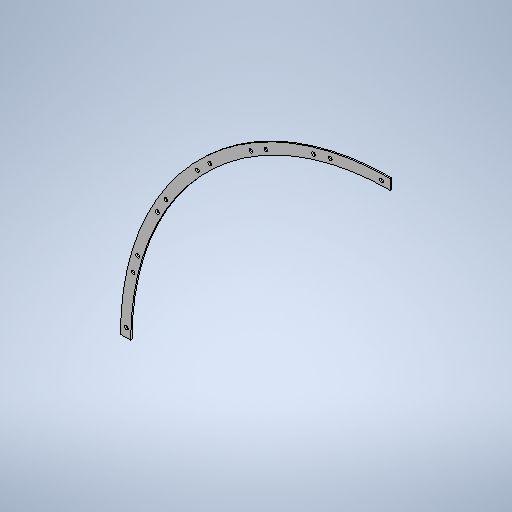
# Autodesk Inventor part: DMF 2.1 01 43 Gear rim 3_CPY
Saved by Autodesk Inventor 2026.2 (Build 302298010, 298A)
## iProperties
Created: 2024-04-30
Part Number: DMF 2.1 01 43 Gear rim 3_CPY
Material: Stainless Steel
Document SubType Name: Sheet Metal
Designer: admin
Stock Number: Барабан_Сектор_Усилителя
Mass: 2673.55 g
Surface Area: 3449.14 cm^2
Volume: 334.194 cm^3
Density: 8 g/cm^3
Flat Pattern Width: 58 cm
Flat Pattern Length: 58 cm
Flat Pattern Area: 3364 cm^2
Sheet Metal Rule: Default
Sheet Metal Width: 580,000 mm
Sheet Metal Length: 580,000 mm
Sheet Metal Area: 336400,000 mm^2
Appearance: Default
Author: pokla
Autodesk Inventor part; units mm, degrees
ref_plane "YZ Plane" through (0, 0, 0) normal (1, 0, 0) x (0, 1, 0)
ref_plane "XZ Plane" through (0, 0, 0) normal (0, 1, 0) x (-1, 0, 0)
ref_plane "XY Plane" through (0, 0, 0) normal (0, 0, 1) x (1, 0, 0)
sketch "Sketch1" plane through (0, 0, 0) normal (0, 0, 1) x (1, 0, 0)
  circle A0 centre (0, 0) radius 558
  circle A1 centre (0, 0) radius 580
  line L0 (0, 0) -> (-580, 0)
  line L1 (0, 0) -> (0, 580) construction
  line L2 (0, 0) -> (0, 580)
  circle A2 centre (0, 0) radius 100
  line L3 (197.082, 197.082) -> (278.716, 0)
  line L4 (278.716, 0) -> (197.082, -197.082)
  line L5 (197.082, -197.082) -> (0, -278.716)
  line L6 (0, -278.716) -> (-197.082, -197.082)
  line L7 (-197.082, -197.082) -> (-278.716, 0)
  line L8 (-278.716, 0) -> (-197.082, 197.082)
  line L9 (-197.082, 197.082) -> (0, 278.716)
  line L10 (0, 278.716) -> (197.082, 197.082)
  point P0 (-558, 0)
  point P1 (0, 558)
  point P2 (-100, 0)
  point P3 (0, 100)
  point P4 (0, 278.716)
  point P5 (-278.716, 0)
  dimension "d30" = 90
  dimension "d31" = 1160
  dimension "d32" = 1116
  dimension "d65" = 90
  dimension "d66" = 200
  dimension "d91" = 515
  measures "d30" angle of L2 L0
  measures "d31" diameter of A1
  measures "d32" diameter of A0
  measures "d65" angle of L1 L0
  measures "d66" diameter of A2
  measures "d91" distance between parallel lines of L5 L9
extrude "Plate1" add sketch "Sketch1" against normal blind 3 contours A0 L0 A1 L2 picked at (-572.0249, 22.0563)
sketch "Sketch2" plane through (0, 0, 0) normal (0, 0, 1) x (1, 0, 0)
  circle A0 centre (0, 0) radius 567.5
  arc A1 (0, 580) -> (-580, 0) centre (0, 0) ccw projected
  line L0 (0, 0) -> (0, 580) construction
  line L1 (0, 0) -> (-18.5681, 567.1962) construction
  line L2 (-128.8658, 552.6752) -> (0, 0) construction
  line L3 (0, 0) -> (0, 567.5) construction
  line L4 (0, 0) -> (18.5681, 567.1962) construction
  line L5 (0, 0) -> (128.8658, 552.6752) construction
  line L6 (0, 0) -> (-164.7366, 543.0636) construction
  line L7 (0, 0) -> (-267.5176, 500.4903) construction
  dimension "d34" = 1135
  dimension "d35" = 1.875
  dimension "d36" = 11.25
  dimension "d44" = 1.875
  dimension "d45" = 11.25
  dimension "d49" = 3.75
  dimension "d50" = 11.25
  constraints: 16 end point, 3 coincident, 1 vertical, 9 other
  measures "d35" angle of L0 L1
  measures "d36" angle of L1 L2
  measures "d44" angle of L4 L3
  measures "d45" angle of L5 L4
  measures "d49" angle of L2 L6
  measures "d50" angle of L6 L7
hole "Hole1" at (-18.5681, 567.1962, 0) at (-128.8658, 552.6752, 0) at (128.8658, 552.6752, 0) at (18.5681, 567.1962, 0) at (-164.7366, 543.0636, 0) at (-267.5176, 500.4903, 0) direction (0, 0, -1) diameter 8 end through all
pattern_circular "Circular Pattern1" count 4 over 90 about axis through (0, 0, -10) along (0, 0, 1) of "Hole1"
equation "\"d31\" = Колесо_диам1_ручья_внеш"
equation "\"d91\" = Барабан_размер_по_плоскостям"
equation "\"d44\" = d35"
equation "\"d45\" = d36"
equation "\"d49\" = 2 * d35"
equation "\"d50\" = d36"
equation "\"d42\" = Thickness"
equation "\"d15\" = Thickness"
equation "\"BendRadius\" = Thickness"
equation "\"BendReliefWidth\" = Thickness"
equation "\"BendReliefDepth\" = 0.5 * Thickness"
equation "\"CornerReliefSize\" = 4 * Thickness"
equation "\"MinimumRemnant\" = 2 * Thickness"
equation "\"TransitionRadius\" = BendRadius"
equation "\"JacobiRadiusSize\" = BendRadius"
equation "\"GapSize\" = Thickness"
equation "\"Колесо_диам1_ручья_внеш\" = 1160"
equation "\"Барабан_размер_по_плоскостям\" = 515"
equation "\"Thickness\" = 3"
body "Solid1"
